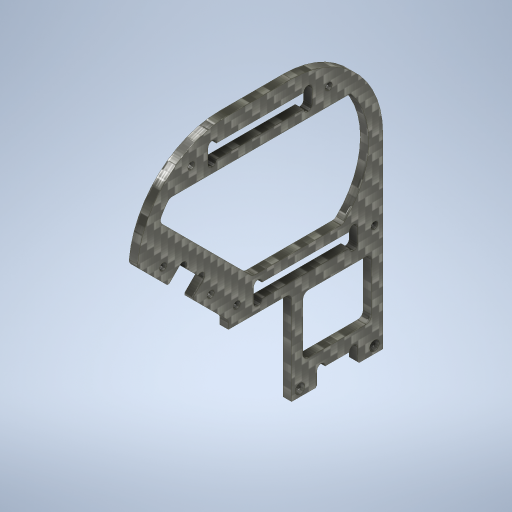
# Autodesk Inventor part: HeadSideFrame
Saved by Autodesk Inventor 2024.2 (Build 282272000, 272)
## iProperties
Created: 2024-06-12
Part Number: HeadSideFrame
Material: CFRP
Document SubType Name: Modeling
Designer: Masato Kubotera
Density: 1.43 g/cm^3
Appearance: Carbon Fiber 1
Author: Masato Kubotera
Autodesk Inventor part; units mm, degrees
ref_plane "YZ Plane" through (0, 0, 0) normal (1, 0, 0) x (0, 1, 0)
ref_plane "XZ Plane" through (0, 0, 0) normal (0, 1, 0) x (-1, 0, 0)
ref_plane "XY Plane" through (0, 0, 0) normal (0, 0, 1) x (1, 0, 0)
sketch "Sketch1" plane through (0, 0, 0) normal (0, 1, 0) x (-1, 0, 0)
  line L0 (-16.25, -1.5) -> (16.25, -1.5)
  line L1 (-7.25, -1.5) -> (-7.25, 3.5) construction
  line L2 (-7.25, 3.5) -> (7.25, 3.5) construction
  line L3 (0, 3.5) -> (0, -1.5) construction
  line L4 (7.25, -1.5) -> (7.25, 3.5) construction
  line L5 (-13.25, 1) -> (13.25, 1) construction
  line L6 (-7.3, -1.5) -> (-7.3, 3.5)
  line L7 (-7.3, 3.5) -> (7.3, 3.5)
  arc A0 (-4.3, 3.5) -> (-7.3, 3.5) centre (-5.8, 3.5) ccw
  line L8 (7.3, -1.5) -> (7.3, 3.5)
  arc A1 (7.3, 3.5) -> (4.3, 3.5) centre (5.8, 3.5) ccw
  line L9 (-16.25, -1.5) -> (-16.25, 32)
  line L10 (16.25, -1.5) -> (16.25, 65)
  ellipse E0 centre (-16.25, 65) end of major axis (18.25, 65) minor radius 35 (-16.25, 30) -> (-16.25, 100) ccw construction
  line L11 (-16.25, 30) -> (-16.25, 100) construction
  line L12 (-16.25, 65) -> (18.25, 65) construction
  ellipse E1 centre (-16.25, 65) end of major axis (16.25, 65) minor radius 33 (-16.25, 32) -> (16.25, 65) ccw construction
  line L13 (-16.25, 32) -> (-38.75, 32)
  line L14 (-16.25, 98) -> (-38.75, 98)
  line L15 (-27.5, 98) -> (-27.5, 32) construction
  ellipse E2 centre (-38.75, 65) end of major axis (-73.25, 65) minor radius 35 (-38.75, 100) -> (-38.75, 30) ccw construction
  ellipse E3 centre (-38.75, 65) end of major axis (-71.25, 65) minor radius 33 (-38.75, 98) -> (-71.1715, 67.2921) ccw
  line L16 (-38.75, 30) -> (-16.25, 30) construction
  line L17 (-38.75, 100) -> (-16.25, 100) construction
  line L18 (-10.25, 30) -> (10.25, 30)
  line L19 (12.25, 28) -> (12.25, 11)
  line L20 (10.25, 9) -> (-10.25, 9)
  line L21 (-12.25, 11) -> (-12.25, 28)
  line L22 (-12.25, 30) -> (12.25, 9) construction
  line L23 (12.25, 30) -> (-12.25, 9) construction
  arc A2 (-10.25, 30) -> (-12.25, 28) centre (-10.25, 28) ccw
  arc A3 (-12.25, 11) -> (-10.25, 9) centre (-10.25, 11) ccw
  arc A4 (10.25, 9) -> (12.25, 11) centre (10.25, 11) ccw
  arc A5 (12.25, 28) -> (10.25, 30) centre (10.25, 28) ccw
  line L24 (-38.75, 30) -> (-38.75, 100) construction
  line L25 (-38.75, 32) -> (-38.75, 34.8706)
  line L26 (-38.75, 34.8706) -> (-71.1715, 67.2921)
  line L27 (-62.0208, 45.9792) -> (-108, 0) construction
  line L28 (-108, 0) -> (0, 0) construction
  ellipse E4 centre (-38.75, 65) end of major axis (-71.25, 65) minor radius 33 (-71.1715, 67.2921) -> (-38.75, 32) ccw construction
  ellipse E5 centre (-16.25, 65) end of major axis (16.25, 65) minor radius 33 (16.25, 65) -> (-16.25, 98) ccw
  line L29 (-55, 91.5815) -> (0, 91.5815) construction
  line L30 (0, 91.5815) -> (0, 86.5815) construction
  line L31 (0, 86.5815) -> (-55, 86.5815) construction
  line L32 (-55, 86.5815) -> (-55, 91.5815) construction
  line L33 (-55, 91.5815) -> (0, 86.5815) construction
  line L34 (0, 91.5815) -> (-55, 86.5815) construction
  line L35 (-47.5, 91.5815) -> (-47.5, 96.7815) construction
  line L36 (-47.5, 96.7815) -> (-7.5, 96.7815) construction
  line L37 (-7.5, 96.7815) -> (-7.5, 91.5815) construction
  line L38 (-46, 91.5815) -> (-46, 86.5815) construction
  line L39 (-52, 89.0815) -> (-3, 89.0815) construction
  line L40 (-9, 91.5815) -> (-9, 86.5815) construction
  line L41 (-8.95, 86.5315) -> (-46.05, 86.5315)
  line L42 (-46.05, 86.5315) -> (-46.05, 91.6315)
  line L43 (-46.05, 91.6315) -> (-8.95, 91.6315)
  line L44 (-8.95, 91.6315) -> (-8.95, 86.5315)
  line L45 (-8.95, 86.5315) -> (-46.05, 91.6315) construction
  line L46 (-46.05, 86.5315) -> (-8.95, 91.6315) construction
  arc A6 (-43.05, 91.6315) -> (-46.05, 91.6315) centre (-44.55, 91.6315) ccw
  arc A7 (-46.05, 86.5315) -> (-43.05, 86.5315) centre (-44.55, 86.5315) ccw
  arc A8 (-8.95, 91.6315) -> (-11.95, 91.6315) centre (-10.45, 91.6315) ccw
  arc A9 (-11.95, 86.5315) -> (-8.95, 86.5315) centre (-10.45, 86.5315) ccw
  line L47 (-54.1012, 75.112) -> (-60.6066, 68.6066) construction
  line L48 (-60.6066, 68.6066) -> (-39.3934, 47.3934) construction
  line L49 (-39.3934, 47.3934) -> (-32.888, 53.8988) construction
  line L50 (-32.888, 53.8988) -> (-54.1012, 75.112) construction
  line L51 (-56.0104, 64.0104) -> (-72.2739, 47.747) construction
  line L52 (-72.2739, 47.747) -> (-60.253, 35.7261) construction
  line L53 (-60.253, 35.7261) -> (-43.9896, 51.9896) construction
  line L54 (-60.1823, 56.3029) -> (-56.0104, 60.4749) construction
  line L55 (-56.0104, 60.4749) -> (-47.5251, 51.9896) construction
  line L56 (-47.5251, 51.9896) -> (-51.6971, 47.8177) construction
  line L57 (-60.2177, 56.3383) -> (-56.0458, 60.5102)
  line L58 (-56.0458, 60.5102) -> (-47.4898, 51.9542)
  line L59 (-47.4898, 51.9542) -> (-51.6617, 47.7823)
  arc A10 (-47.4898, 51.9542) -> (-49.6111, 54.0756) centre (-48.5504, 53.0149) ccw
  arc A11 (-53.9244, 58.3889) -> (-56.0458, 60.5102) centre (-54.9851, 59.4496) ccw
  line L60 (-62.0208, 62.9497) -> (-45.0503, 45.9792) construction
  line L61 (-51.7678, 56.2322) -> (-55.3033, 52.6967) construction
  line L62 (-59.5459, 56.9393) -> (-51.0607, 48.4541) construction
  circle A12 centre (-45.0503, 45.9792) radius 2.4 construction
  circle A13 centre (-45.0503, 45.9792) radius 1.25 construction
  line L63 (-65.9099, 63.3033) -> (-62.3744, 66.8388) construction
  line L64 (-44.6967, 42.0901) -> (-41.1612, 45.6256) construction
  line L65 (-29.75, 40.55) -> (7.25, 40.55) construction
  line L66 (7.25, 40.55) -> (7.25, 35.55) construction
  line L67 (7.25, 35.55) -> (-29.75, 35.55) construction
  line L68 (-29.75, 35.55) -> (-29.75, 40.55) construction
  line L69 (-29.75, 40.55) -> (7.25, 35.55) construction
  line L70 (7.25, 40.55) -> (-29.75, 35.55) construction
  line L71 (-35.75, 38.05) -> (13.25, 38.05) construction
  line L72 (-11.25, 40.55) -> (-11.25, 35.55) construction
  line L73 (-38.75, 40.55) -> (-38.75, 35.55) construction
  line L74 (16.25, 40.55) -> (16.25, 35.55) construction
  line L75 (-29.8, 40.6) -> (7.3, 40.6)
  line L76 (7.3, 40.6) -> (7.3, 35.5)
  line L77 (7.3, 35.5) -> (-29.8, 35.5)
  line L78 (-29.8, 35.5) -> (-29.8, 40.6)
  line L79 (-29.8, 40.6) -> (7.3, 35.5) construction
  line L80 (7.3, 40.6) -> (-29.8, 35.5) construction
  arc A14 (4.3, 35.5) -> (7.3, 35.5) centre (5.8, 35.5) ccw
  arc A15 (7.3, 40.6) -> (4.3, 40.6) centre (5.8, 40.6) ccw
  arc A16 (-29.8, 35.5) -> (-26.8, 35.5) centre (-28.3, 35.5) ccw
  arc A17 (-26.8, 40.6) -> (-29.8, 40.6) centre (-28.3, 40.6) ccw
  line L81 (-59.7893, 83.0315) -> (4.7893, 83.0315)
  line L82 (-63.4241, 77.3638) -> (-30.1603, 44.1)
  ellipse E6 centre (-16.25, 65) end of major axis (11.25, 65) minor radius 28.0012 (2.0513, 44.1) -> (11.25, 65) ccw
  ellipse E7 centre (-16.25, 65) end of major axis (11.25, 65) minor radius 28.0012 (11.25, 65) -> (4.7893, 83.0315) ccw
  ellipse E8 centre (-38.75, 65) end of major axis (-66.25, 65) minor radius 28.0012 (-59.7893, 83.0315) -> (-63.4241, 77.3638) ccw
  line L83 (-16.25, 65) -> (8.5857, 86.2852) construction
  line L84 (-30.1603, 44.1) -> (2.0513, 44.1)
  line L85 (-62.0208, 45.9792) -> (-32.844, 9.9488)
  line L86 (-32.844, 9.9488) -> (-98.0512, 75.156)
  line L87 (-98.0512, 75.156) -> (-62.0208, 45.9792)
  line L88 (-38.75, 65) -> (-73.25, 65) construction
  point P0 (0, 1)
  point P1 (0, 19.5)
  point P2 (5.8, 5)
  point P3 (-27.5, 89.0815)
  point P4 (-53.5355, 54.4645)
  point P5 (-50, 58)
  point P6 (-11.25, 38.05)
  point P7 (-11.25, 38.05)
  point P8 (4.3, 3.5)
  point P9 (-53.9244, 58.3889)
  point P10 (-26.8, 35.5)
  point P11 (-26.8, 40.6)
  point P12 (4.3, 40.6)
  point P13 (-11.95, 91.6315)
  point P14 (-11.95, 86.5315)
  point P15 (-43.05, 86.5315)
  point P16 (-10.45, 85.0315)
  point P17 (-28.3, 34)
  point P18 (5.8, 42.1)
  point P19 (-27.5, 89.0815)
  dimension "d0" = 32.5
  dimension "d1" = 9
  dimension "d2" = 6
  dimension "d3" = 1.5
  dimension "d4" = 5
  dimension "d5" = 0.05
  dimension "d7" = 1.5
  dimension "d8" = 70
  dimension "d10" = 100
  dimension "d12" = 2
  dimension "d14" = 2
  dimension "d15" = 22.5
  dimension "d16" = 4
  dimension "d18" = 2
  dimension "d19" = 55
  dimension "d20" = 5
  dimension "d21" = 5.2
  dimension "d22" = 40
  dimension "d24" = 9
  dimension "d25" = 6
  dimension "d26" = 0.05
  dimension "d27" = 0.05
  dimension "d28" = 6
  dimension "d29" = 9.2
  dimension "d30" = 23
  dimension "d31" = 17
  dimension "d32" = 30
  dimension "d33" = 0.05
  dimension "d34" = 5
  dimension "d35" = 6
  dimension "d36" = 2.5
  dimension "d37" = 4.8
  dimension "d38" = 2.5
  dimension "d39" = 1
  dimension "d40" = 50
  dimension "d41" = 58
  dimension "d42" = 45
  dimension "d43" = 30
  dimension "d44" = 9
  dimension "d46" = 5
  dimension "d47" = 6
  dimension "d48" = 9
  dimension "d49" = 0.05
  dimension "d50" = 0.05
  dimension "d54" = 5
  dimension "d56" = 10
  dimension "d59" = 5
  dimension "d61" = 3.55
  dimension "d80" = 55
  dimension "d83" = 2
  dimension "d84" = 2
  dimension "d85" = 168
  dimension "d86" = 24.5
  dimension "d87" = 2
  constraints: 178 end point, 43 point on line, 36 point on circle, 36 symmetric about line, 27 midpoint, 22 horizontal, 18 centre point, 16 parallel, 14 coincident, 13 perpendicular, 13 vertical, 8 tangent, 6 equal radius, 5 collinear, 55 other
  measures "d0" distance of L0.start L0.end
  measures "d1" distance of L0.end L4.start
  measures "d2" distance from line of point (13.25, 1) L4
  measures "d3" distance of L3.end L28.end
  measures "d4" distance from line of L4.start L2
  measures "d5" distance between parallel lines of L6 L1
  measures "d7" radius of A0
  measures "d8" distance of L11.start L11.end
  measures "d10" vertical distance of L28.end L11.end
  measures "d12" distance of L12.end L10.end
  measures "d14" distance of L11.start L9.end
  measures "d15" distance of point (-16.25, 65) point (-38.75, 65)
  measures "d16" distance from line of point (5.8, 5) L20
  measures "d18" radius of A2
  measures "d19" distance of L30.end L31.end
  measures "d20" distance of L29.end L30.end
  measures "d21" distance of L35.start L35.end
  measures "d22" distance of L35.end L36.end
  measures "d24" distance between parallel lines of L38 L32
  measures "d25" distance from line of L38 L39.start
  measures "d26" distance between parallel lines of L29 L43
  measures "d27" distance between parallel lines of L42 L38
  measures "d28" distance from line of L52 L85.start
  measures "d29" distance of L48.end L49.end
  measures "d30" distance between parallel lines of L52 L48
  measures "d31" distance of L51.end L52.end
  measures "d32" distance of L47.end L48.end
  measures "d33" distance between parallel lines of L59 L56
  measures "d34" distance between parallel lines of L62 L55
  measures "d35" distance from line of point (-45.05, 45.979) L56
  measures "d36" distance between parallel lines of L55 L48
  measures "d37" diameter of A12
  measures "d38" diameter of A13
  measures "d39" distance edge to line of A12 L26
  measures "d40" horizontal distance of L28.end point (-50, 58)
  measures "d41" vertical distance of L28.end point (-50, 58)
  measures "d42" angle of L28 L27
  measures "d43" distance between parallel lines of L64 L63
  measures "d44" distance between parallel lines of L63 L54
  measures "d46" distance of L65.end L66.end
  measures "d47" distance from line of point (-35.75, 38.05) L68
  measures "d48" distance between parallel lines of L73 L68
  measures "d49" distance between parallel lines of L76 L66
  measures "d50" distance between parallel lines of L77 L67
  measures "d54" distance of point (11.25, 65) L10.end
  measures "d56" diameter of L82 L50
  measures "d59" distance of L83.end L81.end
  measures "d61" distance between parallel lines of L81 L31
  measures "d80" horizontal distance of L0.end L16.start
  measures "d83" distance from line of point (-28.3, 34) L13
  measures "d84" distance from line of point (5.8, 42.1) L84
  measures "d85" angle of L87 L85
  measures "d86" distance between parallel lines of L19 L21
  measures "d87" distance from line of point (-10.45, 85.031) L81
extrude "Extrusion1" add sketch "Sketch1" along normal blind 3 contours L9 L13 L25 L26 L59 A10 L58 A11 L57 E3 L14 E5 L10 L0 L8 A1 L7 A0 L6
hole "Phi3.5" at (13.25, 0, 1) at (-13.25, 0, 1) direction (0, 1, 0) diameter 3.5 end through all
hole "Phi2.5" at (52, 0, 89.0815) at (3, 0, 89.0815) at (62.0208, 0, 62.9497) at (45.0503, 0, 45.9792) at (35.75, 0, 38.05) at (-13.25, 0, 38.05) direction (0, 1, 0) diameter 2.5 end through all
chamfer "C0.5" distance 0.5 angle 45 4 edges at (60.2177, 1.5, 56.3383) (51.6617, 1.5, 47.7823) (7.3, 1.5, -1.5) (-7.3, 1.5, -1.5)
fillet "R2" radius 2 8 edges at (63.4241, 1.5, 77.3638) (59.7893, 1.5, 83.0315) (-4.7893, 1.5, 83.0315) (-2.0513, 1.5, 44.1) (30.1603, 1.5, 44.1) (16.25, 1.5, 32) (38.75, 1.5, 34.8706) (71.1715, 1.5, 67.2921)
equation "\"d14\" = d12"
body "Solid1"
